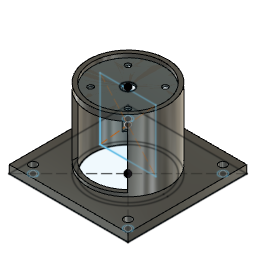
base-braco-robotico (Autodesk Fusion 360 design; units mm, degrees)
Autodesk Fusion 360 part; units mm, degrees
note: some values were not read from the file. Set by a fixed rule: which sketch regions a step uses.
sketch "Sketch1" plane through (0, 0, 0) normal (0, 0, 1) x (1, 0, 0)
  line L0 (75, 75) -> (-75, 75)
  line L1 (-75, 75) -> (-75, -75)
  line L2 (-75, -75) -> (75, -75)
  line L3 (75, -75) -> (75, 75)
  line L4 (75, 75) -> (-75, -75) construction
  line L5 (-75, 75) -> (75, -75) construction
  circle A0 centre (-60, 60) radius 5
  circle A1 centre (60, 60) radius 5
  circle A2 centre (-60, -60) radius 5
  circle A3 centre (60, -60) radius 5
  circle A4 centre (0, 0) radius 50
  circle A5 centre (0, 0) radius 45
  dimension "d1" = 150
  dimension "d2" = 150
  dimension "d3" = 10
  dimension "d4" = 10
  dimension "d5" = 10
  dimension "d6" = 10
  dimension "d7" = 100
  dimension "d8" = 90
  constraint horizontal L0
  constraint perpendicular L0 L1
  constraint parallel L0 L2
  constraint parallel L1 L3
  constraint coincident L4 A4.centre
  constraint coincident L5 A4.centre
  constraint coincident A4.centre A5.centre
  constraint coincident L5 A0.centre
  constraint coincident L4 A1.centre
  constraint coincident L4 A2.centre
  constraint coincident L5 A3.centre
  measures "d1" distance of L1.end L2.end
  measures "d2" distance of L0 L2
  measures "d3" diameter of A0
  measures "d4" diameter of A1
  measures "d5" diameter of A2
  measures "d6" diameter of A3
  measures "d7" diameter of A4
  measures "d8" diameter of A5
extrude "Extrude1" add sketch "Sketch1" along normal blind 10 contours L0 L1 L2 L3
extrude "Extrude2" add sketch "Sketch1" along normal blind 100 contours A4
extrude "Extrude3" add sketch "Sketch1" along normal blind 95 contours A5
extrude "Extrude4" cut sketch "Sketch1" along normal blind 90 contours A5
sketch "Sketch2" plane through (0, 0, 95) normal (0, 0, 1) x (-1, 0, 0)
  circle A0 centre (0, 0) radius 45
  circle A1 centre (0, 0) radius 7.5
  dimension "d17" = 15
  constraint coincident A0.centre A1.centre
  measures "d17" diameter of A1
extrude "Extrude5" cut sketch "Sketch2" against normal blind 10 contours A1
sketch "Sketch3" plane through (0, 0, 0) normal (0, 1, 0) x (1, 0, 0)
  line L0 (35.1024, -92.6698) -> (-35.2945, -92.6698)
  line L1 (-35.2945, -92.6698) -> (-35.2945, -14.3779)
  line L2 (-35.2945, -14.3779) -> (35.1024, -14.3779)
  line L3 (35.1024, -14.3779) -> (35.1024, -92.6698)
  line L4 (35.1024, -92.6698) -> (-35.2945, -14.3779) construction
  line L5 (-35.2945, -92.6698) -> (35.1024, -14.3779) construction
  point P0 (-0.096, -53.5238)
  constraint horizontal L0
  constraint perpendicular L0 L1
  constraint parallel L0 L2
  constraint parallel L1 L3
  constraint coincident L4 P0
  constraint coincident L5 P0
extrude "Extrude6" cut sketch "Sketch3" along normal mid plane 120
sketch "Sketch4" plane through (0, 0, 95) normal (0, 0, 1) x (-1, 0, 0)
  line L0 (23.622, 23.622) -> (-23.622, 23.622)
  line L1 (-23.622, 23.622) -> (-23.622, -23.622)
  line L2 (-23.622, -23.622) -> (23.622, -23.622)
  line L3 (23.622, -23.622) -> (23.622, 23.622)
  line L4 (23.622, 23.622) -> (-23.622, -23.622) construction
  line L5 (-23.622, 23.622) -> (23.622, -23.622) construction
  circle A0 centre (23.622, 23.622) radius 3.5
  circle A1 centre (-23.622, 23.622) radius 3.5
  circle A2 centre (23.622, -23.622) radius 3.5
  circle A3 centre (-23.622, -23.622) radius 3.5
  dimension "d22" = 47.244
  dimension "d23" = 47.244
  dimension "d24" = 7
  dimension "d25" = 7
  dimension "d26" = 7
  dimension "d27" = 7
  constraint horizontal L0
  constraint perpendicular L0 L1
  constraint parallel L0 L2
  constraint parallel L1 L3
  constraint coincident L4 origin
  constraint coincident L5 origin
  constraint coincident L0.start L3.end
  constraint coincident L0.end L1.start
  constraint coincident L2.end L3.start
  constraint coincident L1.end L2.start
  measures "d22" distance of L1.end L2.end
  measures "d23" distance of L0 L2
  measures "d24" diameter of A0
  measures "d25" diameter of A1
  measures "d26" diameter of A2
  measures "d27" diameter of A3
extrude "Extrude7" cut sketch "Sketch4" against normal blind 10 contours L0 L1 A1 | L0 L1 A1 | L0 L3 A0 | L0 L3 A0 | L1 L2 A3 | L1 L2 A3 | L2 L3 A2 | L2 L3 A2
